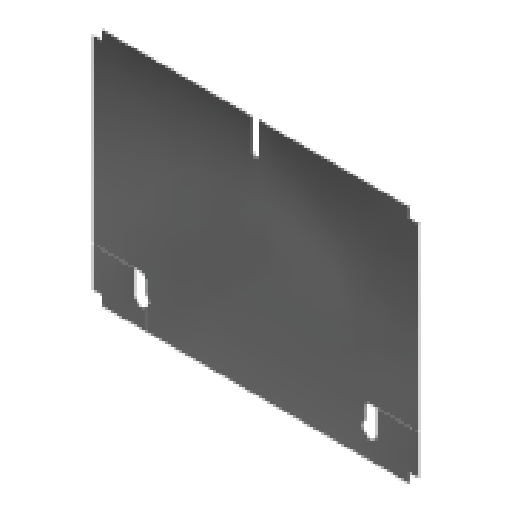
# Autodesk Inventor part: Electronics Cover
Saved by Autodesk Inventor 2023.2 (Build 272271000, 271)
## iProperties
Created: 2023-02-06
Part Number: Electronics Cover
Material: Aluminum 6061
Document SubType Name: Modeling
Designer: remop
Density: 2.7 g/cm^3
Appearance: Aluminum - Flat
Author: remop
Autodesk Inventor part; units mm, degrees
ref_plane "YZ Plane" through (0, 0, 0) normal (1, 0, 0) x (0, 1, 0)
ref_plane "XZ Plane" through (0, 0, 0) normal (0, 1, 0) x (-1, 0, 0)
ref_plane "XY Plane" through (0, 0, 0) normal (0, 0, 1) x (1, 0, 0)
sketch "Sketch1" plane through (0, 0, 0) normal (0, 0, 1) x (1, 0, 0)
  line L0 (500, 375) -> (0, 375) projected
  line L1 (-15, 0) -> (-15, 360) projected
  line L2 (0, 0) -> (0, 360) projected
  line L3 (515, 0) -> (515, 360) projected
  line L4 (0, 0) -> (500, 0) projected
  line L5 (500, 0) -> (500, 360) projected
  line L6 (500, 360) -> (0, 360) projected
  line L7 (0, -15) -> (500, -15) projected
  line L8 (-15, 359.5) -> (0, 359.5)
  line L9 (0.5, 360) -> (0.5, 375)
  line L10 (0, 0.5) -> (-15, 0.5)
  line L11 (0.5, 0) -> (0.5, -15)
  line L12 (499.5, 375) -> (499.5, 360)
  line L13 (500, 359.5) -> (515, 359.5)
  line L14 (499.5, 0) -> (499.5, -15)
  line L15 (500, 0.5) -> (515, 0.5)
  line L16 (350, 375) -> (350, -15)
  line L17 (349.5, -15) -> (349.5, 375)
  line L18 (150, 375) -> (150, -15)
  line L19 (150.5, -15) -> (150.5, 375)
  circle A0 centre (250, 324) radius 3 projected
  circle A1 centre (250, 324) radius 5
  line L20 (245, 324) -> (245, 375)
  line L21 (255, 324) -> (255, 375)
  circle A2 centre (436, 58) radius 3 projected
  circle A3 centre (64, 58) radius 3 projected
  circle A4 centre (64, 58) radius 7.5
  circle A5 centre (436, 58) radius 7.5
  line L22 (64, 65.5) -> (-15, 65.5)
  line L23 (71.5, 58) -> (71.5, -15)
  line L24 (428.5, 58) -> (428.5, -15)
  line L25 (436, 65.5) -> (515, 65.5)
  circle A6 centre (436, 28) radius 6 projected
  circle A7 centre (64, 28) radius 6 projected
  circle A8 centre (64, 28) radius 12.5
  circle A9 centre (436, 28) radius 12.5
  line L26 (0.5, 360) -> (0.5, 359.5)
  line L27 (0.5, 359.5) -> (0, 359.5)
  line L28 (499.5, 360) -> (499.5, 359.5)
  line L29 (499.5, 359.5) -> (500, 359.5)
  line L30 (0, 0.5) -> (0.5, 0.5)
  line L31 (0.5, 0.5) -> (0.5, 0)
  line L32 (500, 0.5) -> (499.5, 0.5)
  line L33 (499.5, 0.5) -> (499.5, 0)
  line L34 (71, 17.6438) -> (71, -15)
  line L35 (51.5, 28) -> (51.5, 65)
  line L36 (51.5, 65) -> (-15, 65)
  line L37 (429, 17.6438) -> (429, -15)
  line L38 (448.5, 28) -> (448.5, 65)
  line L39 (448.5, 65) -> (515, 65)
  point P0 (0, 65.5)
  point P1 (71.5, 0)
  point P2 (428.5, 0)
  point P3 (500, 65.5)
  point P4 (350, 360)
  point P5 (350, 0)
  point P6 (255, 360)
  point P7 (245, 360)
  point P8 (150.5, 360)
  point P9 (150.5, 0)
  point P10 (349.5, 0)
  point P11 (349.5, 360)
  point P12 (150, 0)
  point P13 (150, 360)
  point P14 (71.5, 38)
  point P15 (71.5, 18)
  point P16 (428.5, 18)
  point P17 (428.5, 38)
  dimension "d0" = 0.5
  dimension "d1" = 0.5
  dimension "d2" = 0.5
  dimension "d3" = 0.5
  dimension "d4" = 0.5
  dimension "d5" = 0.5
  dimension "d6" = 0.5
  dimension "d7" = 0.5
  dimension "d8" = 0.5
  dimension "d9" = 0.5
  dimension "d10" = 150
  dimension "d11" = 150
  dimension "d12" = 10
  dimension "d13" = 15
  dimension "d16" = 25
  dimension "d18" = 0.5
  dimension "d19" = 0.5
  dimension "d20" = 0.5
  dimension "d21" = 0.5
  constraints: 64 end point, 27 point on line, 19 perpendicular, 10 point on circle, 10 vertical, 6 tangent, 5 centre point, 5 coincident, 2 equal radius, 1 horizontal, 20 other
  measures "d0" distance from line of point (0, 375) L9
  measures "d1" distance from line of L2.end L8
  measures "d2" distance between parallel lines of L4 L10
  measures "d3" distance between parallel lines of L2 L11
  measures "d4" distance between parallel lines of L12 L5
  measures "d5" distance between parallel lines of L6 L13
  measures "d6" distance between parallel lines of L4 L15
  measures "d7" distance between parallel lines of L5 L14
  measures "d8" distance between parallel lines of L19 L18
  measures "d9" distance between parallel lines of L16 L17
  measures "d10" distance between parallel lines of L2 L18
  measures "d11" distance between parallel lines of L5 L16
  measures "d12" diameter of A1
  measures "d13" diameter of A4
  measures "d16" diameter of A8
  measures "d18" distance between parallel lines of L34 L23
  measures "d19" distance between parallel lines of L22 L36
  measures "d20" distance between parallel lines of L24 L37
  measures "d21" distance between parallel lines of L25 L39
extrude "Extrusion1" add sketch "Sketch1" along normal blind 2 contours L12 L6 L16 L0 | L28 L29 L5 L25 A5 L24 A9 L4 L16 L6 | L17 L6 L21 L0 | L17 L4 L19 L6 L20 A1 L21 | L4 L24 L7 L16 | L13 L3 L25 L5 | L20 L6 L19 L0 | L17 L7 L19 L4 | L37 A9 L38 L39 L5 L32 L33 L4 | L4 L14 L7 L37 | L39 L3 L15 L5 | L18 L6 L9 L0 | L18 L7 L23 L4 | L4 L23 A8 A4 L22 L2 L27 L26 L6 L18 | L34 L7 L11 L4 | L4 L31 L30 L2 L36 L35 A8 L34 | L2 L22 L1 L8 | L10 L1 L36 L2
fillet "Fillet1" radius 2 14 edges at (71.5, 38, 1) (71.5, 18, 1) (428.5, 18, 1) (428.5, 38, 1) (428.5, -15, 1) (515, 65.5, 1) (515, 359.5, 1) (499.5, 375, 1) (71.5, -15, 1) (-15, 65.5, 1) (0.5, 375, 1) (-15, 359.5, 1) (255, 375, 1) (245, 375, 1)
equation "\"d1\" = d0"
equation "\"d2\" = d0"
equation "\"d3\" = d0"
equation "\"d4\" = d0"
equation "\"d5\" = d0"
equation "\"d6\" = d0"
equation "\"d7\" = d0"
equation "\"d8\" = d0"
equation "\"d9\" = d0"
equation "\"d11\" = d10"
equation "\"d19\" = d18"
equation "\"d20\" = d18"
equation "\"d21\" = d20"
body "Solid1"
